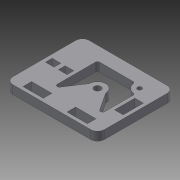
# Autodesk Inventor part: Air2D_Side_Face
Saved by Autodesk Inventor 2014 (Build 180170000, 170)
## iProperties
Created: 2014-09-30
Part Number: Air2D_Side_Face
Material: Generic
Document SubType Name: Modeling
Designer: ThatOtherGuy
Density: 1 g/cm^3
Appearance: Default
Author: ThatOtherGuy
Autodesk Inventor part; units mm, degrees
ref_plane "YZ Plane" through (0, 0, 0) normal (1, 0, 0) x (0, 1, 0)
ref_plane "XZ Plane" through (0, 0, 0) normal (0, 1, 0) x (-1, 0, 0)
ref_plane "XY Plane" through (0, 0, 0) normal (0, 0, 1) x (1, 0, 0)
sketch "Sketch1" plane through (0, 0, 0) normal (0, 0, 1) x (1, 0, 0)
  circle A0 centre (0, 0) radius 2.5
  circle A1 centre (15.5, 15.5) radius 1.6
  line L0 (-19.231, 2.5) -> (-12.5, 2.5)
  line L1 (-12.5, 2.5) -> (-12.5, -2.5)
  line L2 (-12.5, -2.5) -> (-19.231, -2.5)
  line L3 (-19.231, -2.5) -> (-19.231, 2.5)
  line L4 (20, 7.5) -> (26.731, 7.5)
  line L5 (26.731, 7.5) -> (26.731, -7.5)
  line L6 (26.731, -7.5) -> (20, -7.5)
  line L7 (20, -7.5) -> (20, 7.5)
  line L8 (-30.769, 27.5) -> (29.231, 27.5)
  line L9 (29.231, 27.5) -> (29.231, -29.231)
  line L10 (29.231, -29.231) -> (-30.769, -29.231)
  line L11 (-30.769, -29.231) -> (-30.769, 27.5)
  line L12 (4.231, -20) -> (19.231, -20)
  line L13 (19.231, -20) -> (19.231, -26.731)
  line L14 (19.231, -26.731) -> (4.231, -26.731)
  line L15 (4.231, -26.731) -> (4.231, -20)
  line L16 (-29.162, 2.5) -> (-22.431, 2.5)
  line L17 (-22.431, 2.5) -> (-22.431, -2.5)
  line L18 (-22.431, -2.5) -> (-29.162, -2.5)
  line L19 (-29.162, -2.5) -> (-29.162, 2.5)
  line L20 (-20.769, -20) -> (-5.769, -20)
  line L21 (-5.769, -20) -> (-5.769, -26.731)
  line L22 (-5.769, -26.731) -> (-20.769, -26.731)
  line L23 (-20.769, -26.731) -> (-20.769, -20)
  line L24 (-10, -17.5) -> (-10, 17.5)
  line L25 (-10, 17.5) -> (10, 17.5)
  line L26 (-10, -17.5) -> (17.5, -17.5)
  line L27 (17.5, -17.5) -> (17.5, 10)
  arc A2 (10, 17.5) -> (17.5, 10) centre (17.5, 17.5) ccw
  line L28 (-10, -17.5) -> (-6, 0)
  line L29 (6, 0) -> (17.5, -17.5)
  arc A3 (6, 0) -> (-6, 0) centre (0, 0) ccw
  circle A4 centre (-15.5, -15.5) radius 1.6
  point P0 (-12.5, 0)
  point P1 (20, 0)
  dimension "d0" = 5
  dimension "d6" = 32.5
  dimension "d7" = 20
  dimension "d8" = 5
  dimension "d9" = 6.731
  dimension "d13" = 20
  dimension "d17" = 2.5
  dimension "d18" = 20
  dimension "d19" = 2.5
  dimension "d20" = 3.2
  dimension "d25" = 15
  dimension "d26" = 10
  dimension "d28" = 60
  dimension "d29" = 10
  dimension "d30" = 15.5
  dimension "d31" = 15.5
  dimension "d32" = 3.2
  dimension "d33" = 2.5
  dimension "d34" = 2.5
  dimension "d35" = 2.5
  dimension "d36" = 7.5
  dimension "d37" = 6
  dimension "d39" = 35
  dimension "d40" = 15.5
  dimension "d41" = 15.5
  constraints: 60 end point, 14 parallel, 8 perpendicular, 7 equal length, 6 horizontal, 5 centre point, 4 coincident, 4 horizontal alignment, 4 point on circle, 2 collinear, 2 line through centre, 2 midpoint, 1 equal radius
  measures "d0" diameter of A0
  measures "d6" distance between parallel lines of L1 L7
  measures "d7" distance from line of L7 point (0, 0)
  measures "d8" distance of L2.end L0.start
  measures "d9" distance of L4.start L4.end
  measures "d13" distance from line of L12 point (0, 0)
  measures "d17" distance between parallel lines of L14 L10
  measures "d18" distance between parallel lines of L4 L8
  measures "d19" distance between parallel lines of L5 L9
  measures "d20" distance between parallel lines of L17 L3
  measures "d25" distance of L6.end L4.start
  measures "d26" distance between parallel lines of L9 L13
  measures "d28" distance of L8.start L8.end
  measures "d29" distance between parallel lines of L11 L23
  measures "d30" horizontal distance of A1.centre point (0, 0)
  measures "d31" horizontal distance of A1.centre point (0, 0)
  measures "d32" diameter of A1
  measures "d33" distance between parallel lines of L7 L27
  measures "d34" distance between parallel lines of L12 L26
  measures "d35" distance between parallel lines of L1 L24
  measures "d36" radius of A2
  measures "d37" radius of A3
  measures "d39" distance of L24.start L24.end
  measures "d40" horizontal distance of point (0, 0) A4.centre
  measures "d41" horizontal distance of point (0, 0) A4.centre
extrude "Extrusion2" add sketch "Sketch1" along normal blind 6.731 contours L8 L9 L10 L11
fillet "Fillet2" radius 5 4 edges at (29.231, 27.5, 3.3655) (29.231, -29.231, 3.3655) (-30.769, -29.231, 3.3655) (-30.769, 27.5, 3.3655)
fillet "Fillet2" radius 1.5875 5 edges at (-10, -17.5, 3.3655) (17.5, -17.5, 3.3655) (17.5, 10, 3.3655) (10, 17.5, 3.3655) (-10, 17.5, 3.3655)
equation "\"d9\" = THICKB"
equation "\"d13\" = d7"
equation "\"d29\" = d26"
equation "\"d30\" = d31"
equation "\"d40\" = d31"
equation "\"d41\" = d31"
equation "\"d22\" = THICKB"
equation "\"THICKA\" = 3.175"
equation "\"THICKB\" = 6.731"
equation "\"THICKC\" = 12.7"
equation "\"BALLDIA\" = 12"
equation "\"MAGDIA\" = 9.5"
body "Solid2"
